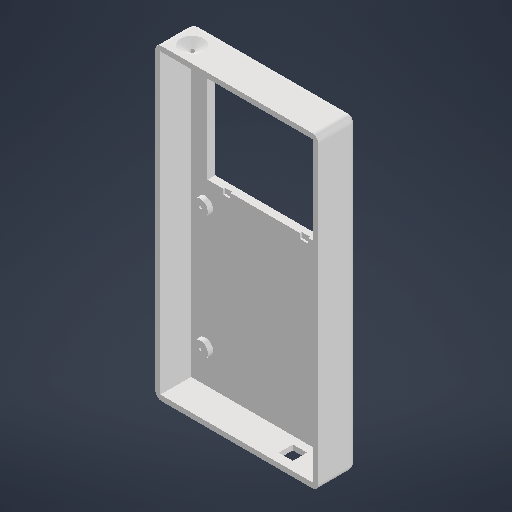
# Autodesk Inventor part: Bottom_Shell
Saved by Autodesk Inventor 2027 (Build 310192000, 192)
## iProperties
Created: 2026-03-03
Part Number: Bottom_Shell
Material: Generic
Document SubType Name: Modeling
Designer: kjedr
Density: 1 g/cm^3
Appearance: Default
Author: kjedr
Autodesk Inventor part; units mm, degrees
ref_plane "YZ Plane" through (0, 0, 0) normal (1, 0, 0) x (0, 1, 0)
ref_plane "XZ Plane" through (0, 0, 0) normal (0, 1, 0) x (-1, 0, 0)
ref_plane "XY Plane" through (0, 0, 0) normal (0, 0, 1) x (1, 0, 0)
sketch "Sketch1" plane through (0, 0, 0) normal (0, 0, 1) x (1, 0, 0)
  line L0 (0, 0) -> (80.8355, 0)
  line L1 (80.8355, 0) -> (80.8355, 152.4)
  line L2 (80.8355, 152.4) -> (0, 152.4)
  line L3 (0, 152.4) -> (0, 0)
  dimension "d82" = 80.8355
  dimension "d90" = 152.4
  constraints: 8 end point, 3 perpendicular
  measures "d82" distance of L1.end L2.end
  measures "d90" distance of L2.end L0.start
extrude "Extrusion1" add sketch "Sketch1" along normal blind 19.05
sketch "Sketch2" plane through (0, 0, 19.05) normal (0, 0, 1) x (1, 0, 0)
  line L0 (2.54, 2.54) -> (78.2955, 2.54)
  line L1 (78.2955, 2.54) -> (78.2955, 149.86)
  line L2 (78.2955, 149.86) -> (2.54, 149.86)
  line L3 (2.54, 149.86) -> (2.54, 2.54)
  line L4 (0, 152.4) -> (0, 0)
  line L5 (0, 0) -> (80.8355, 0)
  line L6 (80.8355, 0) -> (80.8355, 152.4)
  line L7 (80.8355, 152.4) -> (0, 152.4)
  line L8 (0, 152.4) -> (0, 0) projected
  line L9 (0, 0) -> (80.8355, 0) projected
  point P0 (80.8355, 76.2)
  point P1 (0, 76.2)
  point P2 (40.4177, 0)
  dimension "d83" = 152.4
  dimension "d85" = 80.8355
  dimension "d86" = 2.54
  dimension "d87" = 2.54
  dimension "d88" = 2.54
  dimension "d89" = 2.54
  constraints: 16 end point, 5 midpoint, 5 perpendicular
  measures "d83" distance of L4.start L4.end
  measures "d85" distance of L6.end L4.start
  measures "d86" horizontal distance of L2.end L4.start
  measures "d87" horizontal distance of L2.end L4.start
  measures "d88" horizontal distance of L4.end L0.start
  measures "d89" horizontal distance of L5.end L0.end
extrude "Extrusion2" cut sketch "Sketch2" against normal blind 15.24 contours L3 L2 L1 L0
fillet "Fillet1" radius 3.175 8 edges at (40.4177, 152.4, 0) (80.8355, 76.2, 0) (80.8355, 0, 9.525) (0, 76.2, 0) (40.4177, 0, 0) (80.8355, 152.4, 9.525) (0, 152.4, 9.525) (0, 0, 9.525)
sketch "Sketch6" plane through (0, 0, 3.81) normal (0, 0, 1) x (1, 0, 0)
  line L0 (5.1487, 87.2258) -> (75.6867, 87.2258) construction
  line L1 (75.6867, 87.2258) -> (75.6867, 3.2258) construction
  line L2 (75.6867, 3.2258) -> (5.1487, 3.2258) construction
  line L3 (5.1487, 3.2258) -> (5.1487, 87.2258) construction
  circle A0 centre (9.6205, 79.9318) radius 1.6 construction
  circle A1 centre (71.2409, 79.9318) radius 1.6 construction
  circle A2 centre (9.6205, 19.2258) radius 1.6 construction
  circle A3 centre (71.2409, 19.2258) radius 1.6 construction
  line L4 (2.54, 149.86) -> (78.2955, 149.86) projected
  line L5 (3.175, 0) -> (77.6605, 0) projected
  line L6 (78.2955, 2.54) -> (2.54, 2.54) projected
  circle A4 centre (9.6205, 79.9318) radius 3.81
  circle A5 centre (71.2409, 79.9318) radius 3.81
  circle A6 centre (9.6205, 19.2258) radius 3.81
  circle A7 centre (71.2409, 19.2258) radius 3.81
  point P0 (0, 0)
  point P1 (40.4177, 87.2258)
  point P2 (40.4177, 149.86)
  point P3 (2.54, 2.54)
  point P4 (14.1287, 30.2258)
  point P5 (46.6867, 15.7258)
  point P6 (60.2637, 3.2258)
  point P7 (80.8355, 12.6941)
  dimension "d18" = 70.538
  dimension "d19" = 84
  dimension "d30" = 3.2
  dimension "d31" = 60.706
  dimension "d32" = 61.6204
  dimension "d33" = 16
  dimension "d34" = 4.4458
  dimension "d36" = 0.6858
  dimension "d37" = 27
  dimension "d38" = 8.98
  dimension "d39" = 12.5
  dimension "d40" = 29
  dimension "d41" = 15.423
  dimension "d69" = 7.62
  dimension "d70" = 7.62
  dimension "d71" = 7.62
  dimension "d72" = 7.62
  constraints: 8 centre point, 8 end point, 4 coincident, 3 equal radius, 3 vertical alignment, 2 horizontal alignment, 2 midpoint, 2 parallel, 1 horizontal, 1 perpendicular, 1 point on line, 1 other
  measures "d18" distance of L1.end L2.end
  measures "d19" distance of L0.end L1.end
  measures "d30" diameter of A0
  measures "d31" distance of A2.centre A0.centre
  measures "d32" distance of A3.centre A2.centre
  measures "d33" distance from line of L2 A3.centre
  measures "d34" distance from line of L1 A3.centre
  measures "d37" distance from line of L2 point (14.129, 30.226)
  measures "d38" distance from line of L3 point (14.129, 30.226)
  measures "d39" distance from line of L2 point (46.687, 15.726)
  measures "d40" distance from line of L1 point (46.687, 15.726)
  measures "d41" distance from line of L1 point (60.264, 3.226)
  measures "d69" diameter of A4
  measures "d70" diameter of A5
  measures "d71" diameter of A6
  measures "d72" diameter of A7
sketch "Sketch11" plane through (3.175, 0, 3.175) normal (0, -1, 0) x (1, 0, 0)
  line L0 (77.6605, 0) -> (77.6605, 15.875) projected
  line L1 (53.5801, 11.4375) -> (60.5801, 11.4375)
  line L2 (60.5801, 11.4375) -> (60.5801, 4.4375)
  line L3 (60.5801, 4.4375) -> (53.5801, 4.4375)
  line L4 (53.5801, 4.4375) -> (53.5801, 11.4375)
  line L5 (53.5801, 11.4375) -> (60.5801, 4.4375) construction
  line L6 (60.5801, 11.4375) -> (53.5801, 4.4375) construction
  line L7 (74.4855, 15.875) -> (74.4855, 0) projected
  line L8 (0, 15.875) -> (74.4855, 15.875) projected
  point P0 (-3.175, -3.175)
  point P1 (57.0801, 7.9375)
  point P2 (60.5801, 7.9375)
  point P3 (74.4855, 7.9375)
  point P4 (37.2427, 15.875)
  dimension "d43" = 7
  dimension "d44" = 7
  dimension "d68" = 19.8374
  constraints: 12 end point, 5 midpoint, 2 parallel, 1 horizontal, 1 horizontal alignment, 1 perpendicular
  measures "d43" distance of L2.end L3.end
  measures "d44" distance of L1.end L2.end
  measures "d68" horizontal distance of point (37.243, 15.875) point (57.08, 7.938)
extrude "Extrusion5" cut sketch "Sketch11" against normal up to surface (2.54 mm away)
extrude "Extrusion7" add sketch "Sketch6" along normal blind 2.54
sketch "Sketch15" plane through (9.6205, 79.9318, 6.35) normal (0, 0, 1) x (1, 0, 0)
  circle A0 centre (0, 0) radius 3.81 projected
  circle A1 centre (61.6204, 0) radius 3.81 projected
  circle A2 centre (61.6204, -60.706) radius 3.81 projected
  circle A3 centre (0, -60.706) radius 3.81 projected
  point P0 (-9.6205, -79.9318)
  point P1 (61.6204, -60.706)
  point P2 (0, -60.706)
  constraints: 4 coincident
hole "Hole3" at (9.6205, 79.9318, 6.35) at (71.2409, 79.9318, 6.35) at (71.2409, 19.2258, 6.35) at (9.6205, 19.2258, 6.35) direction (0, 0, -1) diameter 1.27 depth 6.35
sketch "Sketch16" plane through (0, 0, 3.81) normal (0, 0, 1) x (1, 0, 0)
  line L0 (10.6608, 140.1387) -> (70.5655, 140.1387)
  line L1 (70.5655, 140.1387) -> (70.5655, 91.2038)
  line L2 (70.5655, 91.2038) -> (10.6608, 91.2038)
  line L3 (10.6608, 91.2038) -> (10.6608, 140.1387)
  point P0 (0, 0)
  constraints: 8 end point, 2 parallel, 1 horizontal, 1 perpendicular
extrude "Extrusion8" cut sketch "Sketch16" against normal blind 25.4
sketch "Sketch17" plane through (2.54, 149.86, 19.05) normal (0, -1, 0) x (1, 0, 0)
  circle A0 centre (7.709, -8.0113) radius 1.27
  point P0 (-2.54, -19.05)
  dimension "d93" = 2.54
  constraints: 1 centre point
  measures "d93" diameter of A0
extrude "Extrusion9" cut sketch "Sketch17" along normal blind 25.4 and the other way blind 12.7 draft 60
sketch "Sketch18" plane through (10.6608, 91.2038, 3.81) normal (0, 1, 0) x (1, 0, 0)
  line L0 (59.9047, 0) -> (0, 0) projected
  line L1 (7.9345, 0) -> (11.287, 0)
  line L2 (11.287, 0) -> (11.287, 0.9229)
  line L3 (11.287, 0.9229) -> (7.9345, 0.9229)
  line L4 (7.9345, 0.9229) -> (7.9345, 0)
  line L5 (45.7582, 0) -> (49.8968, 0)
  line L6 (49.8968, 0) -> (49.8968, 0.9229)
  line L7 (49.8968, 0.9229) -> (45.7582, 0.9229)
  line L8 (45.7582, 0.9229) -> (45.7582, 0)
  point P0 (-10.6608, 3.81)
  point P1 (11.287, 0)
  constraints: 16 end point, 4 parallel, 3 point on line, 2 horizontal, 2 perpendicular
extrude "Extrusion10" cut sketch "Sketch18" against normal blind 2.54
sketch "Sketch19" plane through (0, 0, 3.81) normal (0, 0, 1) x (1, 0, 0)
  point P0 (0, 0)
sketch "Sketch20" plane through (0, 0, 3.81) normal (0, 0, 1) x (1, 0, 0)
  line L0 (10.6608, 140.1387) -> (70.5655, 140.1387) projected
  line L1 (49.8495, 146.7499) -> (57.4821, 146.7499)
  line L2 (57.4821, 146.7499) -> (57.4821, 140.1387)
  line L3 (57.4821, 140.1387) -> (49.8495, 140.1387)
  line L4 (49.8495, 140.1387) -> (49.8495, 146.7499)
  point P0 (0, 0)
  constraints: 8 end point, 2 parallel, 1 horizontal, 1 perpendicular, 1 point on line
extrude "Extrusion11" add sketch "Sketch20" along normal blind 3.81
sketch "Sketch22" plane through (0, 0, 7.62) normal (0, 0, 1) x (1, 0, 0)
  point P0 (0, 0)
  point P1 (53.6723, 143.6065)
hole "Hole4" at (53.6723, 143.6065, 7.62) direction (0, 0, -1) diameter 2.286 end through all
body "Solid1"
